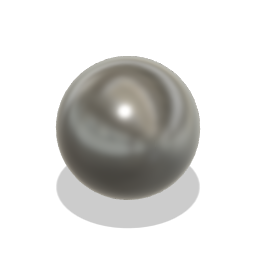
pinball (Autodesk Fusion 360 design; units mm, degrees)
Autodesk Fusion 360 part; units mm, degrees
sphere "SpherePrimitive1" add diameter 26.9875 placed x (1, 0, 0) y (0, 0, -1) z (0, 1, 0) at (0, 0, 0)
equation "d1 = 1 1/16\""
